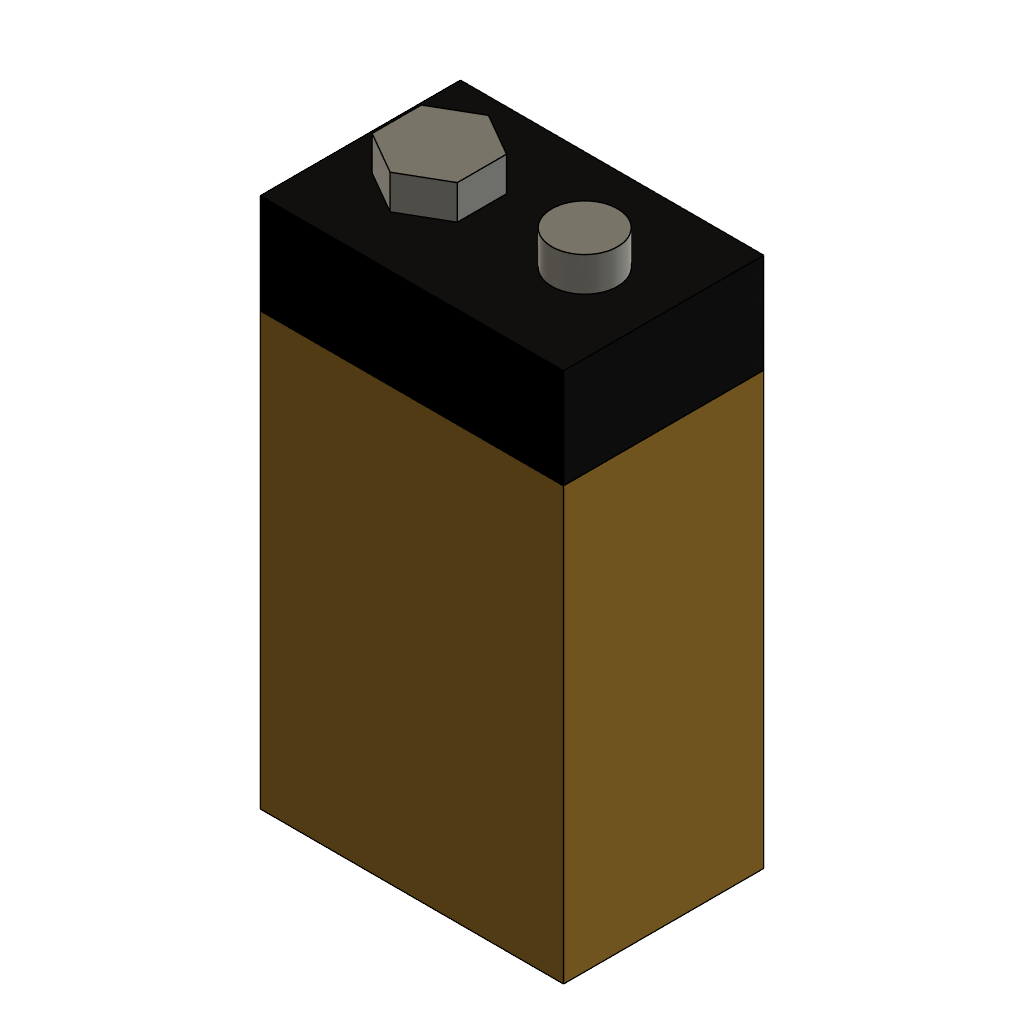
asemblyvol1 (Autodesk Fusion 360 archive; units mm, degrees)
design "battery (9V) 1"
Autodesk Fusion 360 part; units mm, degrees
sketch "Battery base sketch" plane through (0, 0, 0) normal (0, 1, 0) x (1, 0, 0)
  line L0 (13.25, 8.75) -> (-13.25, 8.75)
  line L1 (-13.25, 8.75) -> (-13.25, -8.75)
  line L2 (-13.25, -8.75) -> (13.25, -8.75)
  line L3 (13.25, -8.75) -> (13.25, 8.75)
  line L4 (13.25, 8.75) -> (-13.25, -8.75) construction
  line L5 (-13.25, 8.75) -> (13.25, -8.75) construction
  dimension "d4" = 26.5
  dimension "d5" = 17.5
  constraint horizontal L0
  constraint perpendicular L0 L1
  constraint parallel L0 L2
  constraint parallel L1 L3
  constraint coincident L4 origin
  constraint coincident L5 origin
  measures "d4" distance of L1.end L2.end
  measures "d5" distance of L0.end L1.end
extrude "Extrude1" add sketch "Battery base sketch" along normal blind 46.4 makes body 1
sketch "Socket sketch" plane through (0, 46.4, 0) normal (0, 1, 0) x (-1, 0, 0)
  line L0 (-13.25, 8.75) -> (-13.25, -8.75)
  line L1 (-13.25, -8.75) -> (13.25, -8.75)
  line L2 (13.25, -8.75) -> (13.25, 8.75)
  line L3 (13.25, 8.75) -> (-13.25, 8.75)
  line L4 (0, 0) -> (6.35, 0) construction
  line L5 (6.35, -4.3) -> (10.0739, -2.15)
  line L6 (10.0739, -2.15) -> (10.0739, 2.15)
  line L7 (10.0739, 2.15) -> (6.35, 4.3)
  line L8 (6.35, 4.3) -> (2.6261, 2.15)
  line L9 (2.6261, 2.15) -> (2.6261, -2.15)
  line L10 (2.6261, -2.15) -> (6.35, -4.3)
  line L11 (0, 0) -> (-6.35, 0) construction
  circle A0 centre (-6.35, 0) radius 2.875
  point P0 (6.35, 0)
  dimension "d11" = 6.35
  dimension "d12" = 4.3
  dimension "d13" = 6.35
  dimension "d14" = 5.75
  constraint coincident L4.start L11.start
  constraint perpendicular L0 L4
  constraint coincident P0 L4.end
  constraint perpendicular L0 L11
  constraint coincident L11.end A0.centre
  measures "d11" distance of L4.start P0
  measures "d12" distance of L5.start P0
  measures "d13" distance of L4.start L11.end
  measures "d14" diameter of A0
extrude "Extrude2" add sketch "Socket sketch" along normal blind 3 separate body contours L5 L6 L7 L8 L9 L10 | A0 makes body 2 at (-5.1087, 46.4, -0.7167) makes body 3 at (3.4786, 48.4, -0.1433)
ref_plane "WorkPlane1" through (0, 37.7, 0) normal (0, 1, 0) x (0, 0, 1)
split_face "SplitFace1" 4 faces at (4.4167, 15.4667, -8.75) (-13.25, 30.9333, -2.9167) (-4.4167, 15.4667, 8.75) (13.25, 30.9333, 2.9167) by plane through (0, 37.7, 0) normal (0, 1, 0) on bodies 1
scale "Scale1" factor 0.272378 about (9.225, 46.4, 0) bodies 2 1 3
equation "batteryHeightMax = 46.4 mm"
equation "batteryWidthMax = 26.5 mm"
equation "batteryDepthMax = 17.5 mm"
equation "d4 = batteryWidthMax"
equation "d5 = batteryDepthMax"
equation "d6 = batteryHeightMax"
equation "socketPlusSocketWidth = 5.75 mm"
equation "socketMinSocketWidth = 8.6 mm"
equation "socketMinSocketSideLength = 4 mm"
equation "d11 = ( 12.7 / 2 ) * 1 mm"
equation "d12 = socketMinSocketWidth / 2"
equation "d14 = socketPlusSocketWidth"
named bodies: "Battery body", "Minus terminal", "Plus terminal"
